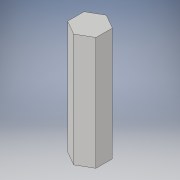
# Autodesk Inventor part: RasPItavt
Saved by Autodesk Inventor 2019 (Build 230136000, 136)
## iProperties
Created: 2019-02-13
Part Number: RasPItavt
Material: Generic
Document SubType Name: Modeling
Designer: izsoandras
Density: 1 g/cm^3
Appearance: Default
Author: izsoandras
Autodesk Inventor part; units mm, degrees
ref_plane "YZ Plane" through (0, 0, 0) normal (1, 0, 0) x (0, 1, 0)
ref_plane "XZ Plane" through (0, 0, 0) normal (0, 1, 0) x (-1, 0, 0)
ref_plane "XY Plane" through (0, 0, 0) normal (0, 0, 1) x (1, 0, 0)
sketch "Sketch1" plane through (0, 0, 0) normal (0, 1, 0) x (-1, 0, 0)
  line L0 (0.6783, 0.1365) -> (-1.8217, 1.5799)
  line L1 (-1.8217, 1.5799) -> (-1.8217, 4.4667)
  line L2 (-1.8217, 4.4667) -> (0.6783, 5.91)
  line L3 (0.6783, 5.91) -> (3.1783, 4.4667)
  line L4 (3.1783, 4.4667) -> (3.1783, 1.5799)
  line L5 (3.1783, 1.5799) -> (0.6783, 0.1365)
  point P0 (0, 0)
  point P1 (0.6783, 3.0233)
  dimension "d0" = 5
  constraints: 12 end point, 13 other
  measures "d0" distance between parallel lines of L1 L4
extrude "Extrusion1" add sketch "Sketch1" along normal blind 20
body "Solid1"
